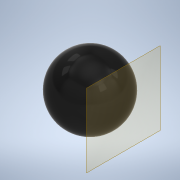
# Autodesk Inventor part: шарик
Saved by Autodesk Inventor 2022 (Build 260153000, 153)
## iProperties
Created: 2021-04-26
Part Number: шарик
Material: Полиацеталь, черный
Document SubType Name: Modeling
Designer: lbfas
Density: 1.425 g/cm^3
Appearance: Гладкая — черная
Author: lbfas
Autodesk Inventor part; units mm, degrees
ref_plane "YZ Plane" through (0, 0, 0) normal (1, 0, 0) x (0, 1, 0)
ref_plane "XZ Plane" through (0, 0, 0) normal (0, 1, 0) x (-1, 0, 0)
ref_plane "XY Plane" through (0, 0, 0) normal (0, 0, 1) x (1, 0, 0)
sketch "Эскиз1" plane through (0, 0, 0) normal (0, 1, 0) x (-1, 0, 0)
  arc A0 (0, -2.5) -> (0, 2.5) centre (0, 0) ccw
  line L0 (0, -4.1922) -> (0, 4.3722)
  dimension "d0" = 5
  constraints: 2 end point, 2 point on circle, 2 point on line, 1 centre point, 1 coincident, 1 vertical
  measures "d0" diameter of A0
revolve "Вращение1" add sketch "Эскиз1" angle 360 about axis through (0, 0, -4.1922) along (0, 0, 1)
